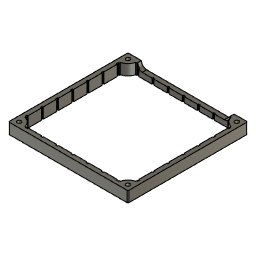
InnerFrame (Autodesk Fusion 360 design; units mm, degrees)
Autodesk Fusion 360 part; units mm, degrees
ref_plane "WorkPlane1" through (0, 0, 36) normal (0, 0, 1) x (1, 0, 0)
sketch "Sketch1" plane through (0, 0, 36) normal (0, 0, 1) x (1, 0, 0)
  line L0 (34, -34) -> (-34, -34)
  line L1 (-34, -34) -> (-34, 34)
  line L2 (-34, 34) -> (34, 34)
  line L3 (34, 34) -> (34, -34)
  line L4 (34, -34) -> (-34, 34) construction
  line L5 (-34, -34) -> (34, 34) construction
  line L6 (-34, 25.5) -> (34, 25.5)
  line L7 (-34, 17) -> (34, 17)
  line L8 (-34, 8.5) -> (34, 8.5)
  line L9 (-34, 0) -> (34, 0)
  line L10 (-25.5, -34) -> (-25.5, 34)
  line L11 (-17, -34) -> (-17, 34)
  line L12 (-8.5, -34) -> (-8.5, 34)
  line L13 (0, -34) -> (0, 34)
  line L14 (-34, 25.5) -> (-25.5, 34) construction
  line L15 (-34, -8.5) -> (34, -8.5)
  line L16 (-34, -17) -> (34, -17)
  line L17 (-34, -25.5) -> (34, -25.5)
  line L18 (-34, -34) -> (34, -34)
  line L19 (8.5, -34) -> (8.5, 34)
  line L20 (17, -34) -> (17, 34)
  line L21 (25.5, -34) -> (25.5, 34)
  line L22 (34, -34) -> (34, 34)
  line L23 (-26.75, 26.75) -> (-32.75, 26.75)
  line L24 (-32.75, 26.75) -> (-32.75, 32.75)
  line L25 (-32.75, 32.75) -> (-26.75, 32.75)
  line L26 (-26.75, 32.75) -> (-26.75, 26.75)
  line L27 (-26.75, 26.75) -> (-32.75, 32.75) construction
  line L28 (-32.75, 26.75) -> (-26.75, 32.75) construction
  line L29 (-24.25, 32.75) -> (-18.25, 32.75)
  line L30 (-24.25, 26.75) -> (-24.25, 32.75)
  line L31 (-18.25, 32.75) -> (-18.25, 26.75)
  line L32 (-18.25, 26.75) -> (-24.25, 26.75)
  line L33 (-15.75, 32.75) -> (-9.75, 32.75)
  line L34 (-15.75, 26.75) -> (-15.75, 32.75)
  line L35 (-9.75, 32.75) -> (-9.75, 26.75)
  line L36 (-9.75, 26.75) -> (-15.75, 26.75)
  line L37 (-7.25, 32.75) -> (-1.25, 32.75)
  line L38 (-7.25, 26.75) -> (-7.25, 32.75)
  line L39 (-1.25, 32.75) -> (-1.25, 26.75)
  line L40 (-1.25, 26.75) -> (-7.25, 26.75)
  line L41 (1.25, 32.75) -> (7.25, 32.75)
  line L42 (1.25, 26.75) -> (1.25, 32.75)
  line L43 (7.25, 32.75) -> (7.25, 26.75)
  line L44 (7.25, 26.75) -> (1.25, 26.75)
  line L45 (9.75, 32.75) -> (15.75, 32.75)
  line L46 (9.75, 26.75) -> (9.75, 32.75)
  line L47 (15.75, 32.75) -> (15.75, 26.75)
  line L48 (15.75, 26.75) -> (9.75, 26.75)
  line L49 (18.25, 32.75) -> (24.25, 32.75)
  line L50 (18.25, 26.75) -> (18.25, 32.75)
  line L51 (24.25, 32.75) -> (24.25, 26.75)
  line L52 (24.25, 26.75) -> (18.25, 26.75)
  line L53 (26.75, 32.75) -> (32.75, 32.75)
  line L54 (26.75, 26.75) -> (26.75, 32.75)
  line L55 (32.75, 32.75) -> (32.75, 26.75)
  line L56 (32.75, 26.75) -> (26.75, 26.75)
  line L57 (-32.75, 24.25) -> (-26.75, 24.25)
  line L58 (-32.75, 18.25) -> (-32.75, 24.25)
  line L59 (-26.75, 24.25) -> (-26.75, 18.25)
  line L60 (-26.75, 18.25) -> (-32.75, 18.25)
  line L61 (-24.25, 24.25) -> (-18.25, 24.25)
  line L62 (-24.25, 18.25) -> (-24.25, 24.25)
  line L63 (-18.25, 24.25) -> (-18.25, 18.25)
  line L64 (-18.25, 18.25) -> (-24.25, 18.25)
  line L65 (-15.75, 24.25) -> (-9.75, 24.25)
  line L66 (-15.75, 18.25) -> (-15.75, 24.25)
  line L67 (-9.75, 24.25) -> (-9.75, 18.25)
  line L68 (-9.75, 18.25) -> (-15.75, 18.25)
  line L69 (-7.25, 24.25) -> (-1.25, 24.25)
  line L70 (-7.25, 18.25) -> (-7.25, 24.25)
  line L71 (-1.25, 24.25) -> (-1.25, 18.25)
  line L72 (-1.25, 18.25) -> (-7.25, 18.25)
  line L73 (1.25, 24.25) -> (7.25, 24.25)
  line L74 (1.25, 18.25) -> (1.25, 24.25)
  line L75 (7.25, 24.25) -> (7.25, 18.25)
  line L76 (7.25, 18.25) -> (1.25, 18.25)
  line L77 (9.75, 24.25) -> (15.75, 24.25)
  line L78 (9.75, 18.25) -> (9.75, 24.25)
  line L79 (15.75, 24.25) -> (15.75, 18.25)
  line L80 (15.75, 18.25) -> (9.75, 18.25)
  line L81 (18.25, 24.25) -> (24.25, 24.25)
  line L82 (18.25, 18.25) -> (18.25, 24.25)
  line L83 (24.25, 24.25) -> (24.25, 18.25)
  line L84 (24.25, 18.25) -> (18.25, 18.25)
  line L85 (26.75, 24.25) -> (32.75, 24.25)
  line L86 (26.75, 18.25) -> (26.75, 24.25)
  line L87 (32.75, 24.25) -> (32.75, 18.25)
  line L88 (32.75, 18.25) -> (26.75, 18.25)
  line L89 (-32.75, 15.75) -> (-26.75, 15.75)
  line L90 (-32.75, 9.75) -> (-32.75, 15.75)
  line L91 (-26.75, 15.75) -> (-26.75, 9.75)
  line L92 (-26.75, 9.75) -> (-32.75, 9.75)
  line L93 (-24.25, 15.75) -> (-18.25, 15.75)
  line L94 (-24.25, 9.75) -> (-24.25, 15.75)
  line L95 (-18.25, 15.75) -> (-18.25, 9.75)
  line L96 (-18.25, 9.75) -> (-24.25, 9.75)
  line L97 (-15.75, 15.75) -> (-9.75, 15.75)
  line L98 (-15.75, 9.75) -> (-15.75, 15.75)
  line L99 (-9.75, 15.75) -> (-9.75, 9.75)
  line L100 (-9.75, 9.75) -> (-15.75, 9.75)
  line L101 (-7.25, 15.75) -> (-1.25, 15.75)
  line L102 (-7.25, 9.75) -> (-7.25, 15.75)
  line L103 (-1.25, 15.75) -> (-1.25, 9.75)
  line L104 (-1.25, 9.75) -> (-7.25, 9.75)
  line L105 (1.25, 15.75) -> (7.25, 15.75)
  line L106 (1.25, 9.75) -> (1.25, 15.75)
  line L107 (7.25, 15.75) -> (7.25, 9.75)
  line L108 (7.25, 9.75) -> (1.25, 9.75)
  line L109 (9.75, 15.75) -> (15.75, 15.75)
  line L110 (9.75, 9.75) -> (9.75, 15.75)
  line L111 (15.75, 15.75) -> (15.75, 9.75)
  line L112 (15.75, 9.75) -> (9.75, 9.75)
  line L113 (18.25, 15.75) -> (24.25, 15.75)
  line L114 (18.25, 9.75) -> (18.25, 15.75)
  line L115 (24.25, 15.75) -> (24.25, 9.75)
  line L116 (24.25, 9.75) -> (18.25, 9.75)
  line L117 (26.75, 15.75) -> (32.75, 15.75)
  line L118 (26.75, 9.75) -> (26.75, 15.75)
  line L119 (32.75, 15.75) -> (32.75, 9.75)
  line L120 (32.75, 9.75) -> (26.75, 9.75)
  line L121 (-32.75, 7.25) -> (-26.75, 7.25)
  line L122 (-32.75, 1.25) -> (-32.75, 7.25)
  line L123 (-26.75, 7.25) -> (-26.75, 1.25)
  line L124 (-26.75, 1.25) -> (-32.75, 1.25)
  line L125 (-24.25, 7.25) -> (-18.25, 7.25)
  line L126 (-24.25, 1.25) -> (-24.25, 7.25)
  line L127 (-18.25, 7.25) -> (-18.25, 1.25)
  line L128 (-18.25, 1.25) -> (-24.25, 1.25)
  line L129 (-15.75, 7.25) -> (-9.75, 7.25)
  line L130 (-15.75, 1.25) -> (-15.75, 7.25)
  line L131 (-9.75, 7.25) -> (-9.75, 1.25)
  line L132 (-9.75, 1.25) -> (-15.75, 1.25)
  line L133 (-7.25, 7.25) -> (-1.25, 7.25)
  line L134 (-7.25, 1.25) -> (-7.25, 7.25)
  line L135 (-1.25, 7.25) -> (-1.25, 1.25)
  line L136 (-1.25, 1.25) -> (-7.25, 1.25)
  line L137 (1.25, 7.25) -> (7.25, 7.25)
  line L138 (1.25, 1.25) -> (1.25, 7.25)
  line L139 (7.25, 7.25) -> (7.25, 1.25)
  line L140 (7.25, 1.25) -> (1.25, 1.25)
  line L141 (9.75, 7.25) -> (15.75, 7.25)
  line L142 (9.75, 1.25) -> (9.75, 7.25)
  line L143 (15.75, 7.25) -> (15.75, 1.25)
  line L144 (15.75, 1.25) -> (9.75, 1.25)
  line L145 (18.25, 7.25) -> (24.25, 7.25)
  line L146 (18.25, 1.25) -> (18.25, 7.25)
  line L147 (24.25, 7.25) -> (24.25, 1.25)
  line L148 (24.25, 1.25) -> (18.25, 1.25)
  line L149 (26.75, 7.25) -> (32.75, 7.25)
  line L150 (26.75, 1.25) -> (26.75, 7.25)
  line L151 (32.75, 7.25) -> (32.75, 1.25)
  line L152 (32.75, 1.25) -> (26.75, 1.25)
  line L153 (-32.75, -1.25) -> (-26.75, -1.25)
  line L154 (-32.75, -7.25) -> (-32.75, -1.25)
  line L155 (-26.75, -1.25) -> (-26.75, -7.25)
  line L156 (-26.75, -7.25) -> (-32.75, -7.25)
  line L157 (-24.25, -1.25) -> (-18.25, -1.25)
  line L158 (-24.25, -7.25) -> (-24.25, -1.25)
  line L159 (-18.25, -1.25) -> (-18.25, -7.25)
  line L160 (-18.25, -7.25) -> (-24.25, -7.25)
  line L161 (-15.75, -1.25) -> (-9.75, -1.25)
  line L162 (-15.75, -7.25) -> (-15.75, -1.25)
  line L163 (-9.75, -1.25) -> (-9.75, -7.25)
  line L164 (-9.75, -7.25) -> (-15.75, -7.25)
  line L165 (-7.25, -1.25) -> (-1.25, -1.25)
  line L166 (-7.25, -7.25) -> (-7.25, -1.25)
  line L167 (-1.25, -1.25) -> (-1.25, -7.25)
  line L168 (-1.25, -7.25) -> (-7.25, -7.25)
  line L169 (1.25, -1.25) -> (7.25, -1.25)
  line L170 (1.25, -7.25) -> (1.25, -1.25)
  line L171 (7.25, -1.25) -> (7.25, -7.25)
  line L172 (7.25, -7.25) -> (1.25, -7.25)
  line L173 (9.75, -1.25) -> (15.75, -1.25)
  line L174 (9.75, -7.25) -> (9.75, -1.25)
  line L175 (15.75, -1.25) -> (15.75, -7.25)
  line L176 (15.75, -7.25) -> (9.75, -7.25)
  line L177 (18.25, -1.25) -> (24.25, -1.25)
  line L178 (18.25, -7.25) -> (18.25, -1.25)
  line L179 (24.25, -1.25) -> (24.25, -7.25)
  line L180 (24.25, -7.25) -> (18.25, -7.25)
  line L181 (26.75, -1.25) -> (32.75, -1.25)
  line L182 (26.75, -7.25) -> (26.75, -1.25)
  line L183 (32.75, -1.25) -> (32.75, -7.25)
  line L184 (32.75, -7.25) -> (26.75, -7.25)
  line L185 (-32.75, -9.75) -> (-26.75, -9.75)
  line L186 (-32.75, -15.75) -> (-32.75, -9.75)
  line L187 (-26.75, -9.75) -> (-26.75, -15.75)
  line L188 (-26.75, -15.75) -> (-32.75, -15.75)
  line L189 (-24.25, -9.75) -> (-18.25, -9.75)
  line L190 (-24.25, -15.75) -> (-24.25, -9.75)
  line L191 (-18.25, -9.75) -> (-18.25, -15.75)
  line L192 (-18.25, -15.75) -> (-24.25, -15.75)
  line L193 (-15.75, -9.75) -> (-9.75, -9.75)
  line L194 (-15.75, -15.75) -> (-15.75, -9.75)
  line L195 (-9.75, -9.75) -> (-9.75, -15.75)
  line L196 (-9.75, -15.75) -> (-15.75, -15.75)
  line L197 (-7.25, -9.75) -> (-1.25, -9.75)
  line L198 (-7.25, -15.75) -> (-7.25, -9.75)
  line L199 (-1.25, -9.75) -> (-1.25, -15.75)
  line L200 (-1.25, -15.75) -> (-7.25, -15.75)
  line L201 (1.25, -9.75) -> (7.25, -9.75)
  line L202 (1.25, -15.75) -> (1.25, -9.75)
  line L203 (7.25, -9.75) -> (7.25, -15.75)
  line L204 (7.25, -15.75) -> (1.25, -15.75)
  line L205 (9.75, -9.75) -> (15.75, -9.75)
  line L206 (9.75, -15.75) -> (9.75, -9.75)
  line L207 (15.75, -9.75) -> (15.75, -15.75)
  line L208 (15.75, -15.75) -> (9.75, -15.75)
  line L209 (18.25, -9.75) -> (24.25, -9.75)
  line L210 (18.25, -15.75) -> (18.25, -9.75)
  line L211 (24.25, -9.75) -> (24.25, -15.75)
  line L212 (24.25, -15.75) -> (18.25, -15.75)
  line L213 (26.75, -9.75) -> (32.75, -9.75)
  line L214 (26.75, -15.75) -> (26.75, -9.75)
  line L215 (32.75, -9.75) -> (32.75, -15.75)
  line L216 (32.75, -15.75) -> (26.75, -15.75)
  line L217 (-32.75, -18.25) -> (-26.75, -18.25)
  line L218 (-32.75, -24.25) -> (-32.75, -18.25)
  line L219 (-26.75, -18.25) -> (-26.75, -24.25)
  line L220 (-26.75, -24.25) -> (-32.75, -24.25)
  line L221 (-24.25, -18.25) -> (-18.25, -18.25)
  line L222 (-24.25, -24.25) -> (-24.25, -18.25)
  line L223 (-18.25, -18.25) -> (-18.25, -24.25)
  line L224 (-18.25, -24.25) -> (-24.25, -24.25)
  line L225 (-15.75, -18.25) -> (-9.75, -18.25)
  line L226 (-15.75, -24.25) -> (-15.75, -18.25)
  line L227 (-9.75, -18.25) -> (-9.75, -24.25)
  line L228 (-9.75, -24.25) -> (-15.75, -24.25)
  line L229 (-7.25, -18.25) -> (-1.25, -18.25)
  line L230 (-7.25, -24.25) -> (-7.25, -18.25)
  line L231 (-1.25, -18.25) -> (-1.25, -24.25)
  line L232 (-1.25, -24.25) -> (-7.25, -24.25)
  line L233 (1.25, -18.25) -> (7.25, -18.25)
  line L234 (1.25, -24.25) -> (1.25, -18.25)
  line L235 (7.25, -18.25) -> (7.25, -24.25)
  line L236 (7.25, -24.25) -> (1.25, -24.25)
  line L237 (9.75, -18.25) -> (15.75, -18.25)
  line L238 (9.75, -24.25) -> (9.75, -18.25)
  line L239 (15.75, -18.25) -> (15.75, -24.25)
  line L240 (15.75, -24.25) -> (9.75, -24.25)
  line L241 (18.25, -18.25) -> (24.25, -18.25)
  line L242 (18.25, -24.25) -> (18.25, -18.25)
  line L243 (24.25, -18.25) -> (24.25, -24.25)
  line L244 (24.25, -24.25) -> (18.25, -24.25)
  line L245 (26.75, -18.25) -> (32.75, -18.25)
  line L246 (26.75, -24.25) -> (26.75, -18.25)
  line L247 (32.75, -18.25) -> (32.75, -24.25)
  line L248 (32.75, -24.25) -> (26.75, -24.25)
  line L249 (-32.75, -26.75) -> (-26.75, -26.75)
  line L250 (-32.75, -32.75) -> (-32.75, -26.75)
  line L251 (-26.75, -26.75) -> (-26.75, -32.75)
  line L252 (-26.75, -32.75) -> (-32.75, -32.75)
  line L253 (-24.25, -26.75) -> (-18.25, -26.75)
  line L254 (-24.25, -32.75) -> (-24.25, -26.75)
  line L255 (-18.25, -26.75) -> (-18.25, -32.75)
  line L256 (-18.25, -32.75) -> (-24.25, -32.75)
  line L257 (-15.75, -26.75) -> (-9.75, -26.75)
  line L258 (-15.75, -32.75) -> (-15.75, -26.75)
  line L259 (-9.75, -26.75) -> (-9.75, -32.75)
  line L260 (-9.75, -32.75) -> (-15.75, -32.75)
  line L261 (-7.25, -26.75) -> (-1.25, -26.75)
  line L262 (-7.25, -32.75) -> (-7.25, -26.75)
  line L263 (-1.25, -26.75) -> (-1.25, -32.75)
  line L264 (-1.25, -32.75) -> (-7.25, -32.75)
  line L265 (1.25, -26.75) -> (7.25, -26.75)
  line L266 (1.25, -32.75) -> (1.25, -26.75)
  line L267 (7.25, -26.75) -> (7.25, -32.75)
  line L268 (7.25, -32.75) -> (1.25, -32.75)
  line L269 (9.75, -26.75) -> (15.75, -26.75)
  line L270 (9.75, -32.75) -> (9.75, -26.75)
  line L271 (15.75, -26.75) -> (15.75, -32.75)
  line L272 (15.75, -32.75) -> (9.75, -32.75)
  line L273 (18.25, -26.75) -> (24.25, -26.75)
  line L274 (18.25, -32.75) -> (18.25, -26.75)
  line L275 (24.25, -26.75) -> (24.25, -32.75)
  line L276 (24.25, -32.75) -> (18.25, -32.75)
  line L277 (26.75, -26.75) -> (32.75, -26.75)
  line L278 (26.75, -32.75) -> (26.75, -26.75)
  line L279 (32.75, -26.75) -> (32.75, -32.75)
  line L280 (32.75, -32.75) -> (26.75, -32.75)
  line L281 (36, -36) -> (-36, -36)
  line L282 (-36, -36) -> (-36, 36)
  line L283 (-36, 36) -> (36, 36)
  line L284 (36, 36) -> (36, -36)
  line L285 (36, -36) -> (-36, 36) construction
  line L286 (-36, -36) -> (36, 36) construction
  line L287 (0.8, -34) -> (0.8, 34)
  line L288 (9.3, -34) -> (9.3, 34)
  line L289 (17.8, -34) -> (17.8, 34)
  line L290 (26.3, -34) -> (26.3, 34)
  line L291 (33.2, 34) -> (33.2, -34)
  line L292 (34.8, 34) -> (34.8, -34)
  line L293 (24.7, -34) -> (24.7, 34)
  line L294 (16.2, -34) -> (16.2, 34)
  line L295 (7.7, -34) -> (7.7, 34)
  line L296 (-0.8, -34) -> (-0.8, 34)
  line L297 (-34, -26.3) -> (34, -26.3)
  line L298 (-34, -24.7) -> (34, -24.7)
  line L299 (-34, -17.8) -> (34, -17.8)
  line L300 (-34, -16.2) -> (34, -16.2)
  line L301 (-34, -9.3) -> (34, -9.3)
  line L302 (-34, -7.7) -> (34, -7.7)
  line L303 (-34, -0.8) -> (34, -0.8)
  line L304 (-34, 0.8) -> (34, 0.8)
  line L305 (-7.7, -34) -> (-7.7, 34)
  line L306 (-9.3, -34) -> (-9.3, 34)
  line L307 (-16.2, -34) -> (-16.2, 34)
  line L308 (-17.8, -34) -> (-17.8, 34)
  line L309 (-24.7, -34) -> (-24.7, 34)
  line L310 (-26.3, -34) -> (-26.3, 34)
  line L311 (-33.2, -34) -> (-33.2, 34)
  line L312 (-34.8, -34) -> (-34.8, 34)
  line L313 (34, -33.2) -> (-34, -33.2)
  line L314 (33.2, -33.2) -> (-33.2, -33.2)
  line L315 (-33.2, -33.2) -> (-33.2, 33.2)
  line L316 (-33.2, 33.2) -> (33.2, 33.2)
  line L317 (33.2, 33.2) -> (33.2, -33.2)
  point P0 (-29.75, 29.75)
  dimension "d701_1_2" = 68
  dimension "d702_1_2" = 68
  dimension "d705_1_2" = 0
  dimension "d706_1_2" = -68
  dimension "d709_1_2" = 68
  dimension "d710_1_2" = 0
  dimension "d711_1_2" = 6
  dimension "d712_1_2" = 6
  dimension "d715_1_2" = 8.5
  dimension "d716_1_2" = -8.5
  dimension "d718_1_2" = 72
  dimension "d719_1_2" = 72
  dimension "d815_2" = 0.8
  dimension "d816_2" = 0.8
  dimension "d817_2" = 0.8
  dimension "d818_2" = 0.8
  dimension "d819_2" = 0.8
  dimension "d825_2" = 0.8
  dimension "d827_2" = 0.8
  dimension "d829_2" = 0.8
  dimension "d831_2" = 0.8
  dimension "d833_2" = 0.8
  dimension "d835_2" = 0.8
  dimension "d837_2" = 0.8
  dimension "d839_2" = 0.8
  dimension "d841_2" = 0.8
  dimension "d1156" = 0.8
  constraint horizontal L0
  constraint perpendicular L0 L1
  constraint parallel L0 L2
  constraint parallel L1 L3
  constraint coincident L4 origin
  constraint coincident L5 origin
  constraint horizontal L23
  constraint perpendicular L23 L24
  constraint parallel L23 L25
  constraint parallel L24 L26
  constraint coincident L27 P0
  constraint coincident L28 P0
  constraint midpoint L14 P0
  constraint horizontal L281
  constraint perpendicular L281 L282
  constraint parallel L281 L283
  constraint parallel L282 L284
  constraint coincident L285 origin
  constraint coincident L286 origin
  measures "d701_1_2" distance of L1.end L2.end
  measures "d702_1_2" distance of L0.end L1.end
  measures "d711_1_2" distance of L24.end L25.end
  measures "d712_1_2" distance of L23.end L24.end
  measures "d718_1_2" distance of L282.end L283.end
  measures "d719_1_2" distance of L281.end L282.end
sketch "Sketch54" plane through (0, 0, 36) normal (0, 0, 1) x (1, 0, 0)
  line L0 (34, -34) -> (-34, -34)
  line L1 (-34, -34) -> (-34, 34)
  line L2 (-34, 34) -> (34, 34)
  line L3 (34, 34) -> (34, -34)
  line L4 (34, -34) -> (-34, 34) construction
  line L5 (-34, -34) -> (34, 34) construction
  line L6 (33.5, -33.5) -> (-33.5, -33.5)
  line L7 (-33.5, -33.5) -> (-33.5, 33.5)
  line L8 (-33.5, 33.5) -> (33.5, 33.5)
  line L9 (33.5, 33.5) -> (33.5, -33.5)
  line L10 (-32.5, -32.5) -> (-32.5, 32.5)
  line L11 (-32.5, 32.5) -> (32.5, 32.5)
  line L12 (32.5, 32.5) -> (32.5, -32.5)
  line L13 (32.5, -32.5) -> (-32.5, -32.5)
  line L14 (-34, 25.5) -> (34, 25.5) construction
  line L15 (-34, 17) -> (34, 17) construction
  line L16 (-34, 8.5) -> (34, 8.5) construction
  line L17 (-34, 0) -> (34, 0) construction
  line L18 (-34, -8.5) -> (34, -8.5) construction
  line L19 (-34, -17) -> (34, -17) construction
  line L20 (-34, -25.5) -> (34, -25.5) construction
  line L21 (-34, -34) -> (34, -34)
  line L22 (-25.5, -34) -> (-25.5, 34) construction
  line L23 (-17, -34) -> (-17, 34) construction
  line L24 (-8.5, -34) -> (-8.5, 34) construction
  line L25 (0, -34) -> (0, 34) construction
  line L26 (8.5, -34) -> (8.5, 34) construction
  line L27 (17, -34) -> (17, 34) construction
  line L28 (25.5, -34) -> (25.5, 34) construction
  line L29 (34, -34) -> (34, 34)
  arc A0 (-26.5, -32.5) -> (-32.5, -26.5) centre (-32.5, -32.5) ccw
  arc A1 (-32.5, 26.5) -> (-26.5, 32.5) centre (-32.5, 32.5) ccw
  arc A2 (26.5, 32.5) -> (32.5, 26.5) centre (32.5, 32.5) ccw
  arc A3 (32.5, -26.5) -> (26.5, -32.5) centre (32.5, -32.5) ccw
  circle A4 centre (-30.5, 30.5) radius 1.1
  circle A5 centre (30.5, 30.5) radius 1.1
  circle A6 centre (-30.5, -30.5) radius 1.1
  circle A7 centre (30.5, -30.5) radius 1.1
  line L30 (-32.5, 17) -> (-32.5, 19)
  line L31 (-31, 19) -> (-31, 0)
  line L32 (-32.5, 17) -> (-32.5, 17.5)
  line L33 (-32.5, 17) -> (-32.5, 16.5)
  line L34 (-32.5, 8.5) -> (-32.5, 9)
  line L35 (-32.5, 8.5) -> (-32.5, 8)
  line L36 (-31, -19) -> (-31, 0)
  line L37 (-19, -31) -> (0, -31)
  line L38 (19, -31) -> (0, -31)
  line L39 (31, -19) -> (31, 0)
  line L40 (31, 19) -> (31, 0)
  line L41 (19, 31) -> (0, 31)
  line L42 (-19, 31) -> (0, 31)
  line L43 (31, 0) -> (31, 0.5)
  line L44 (31, 0) -> (31, -0.5)
  line L45 (31, 19) -> (31, 26.6905)
  line L46 (19, 31) -> (26.6905, 31)
  line L47 (-19, 31) -> (-26.6905, 31)
  line L48 (-31, 19) -> (-31, 26.6905)
  line L49 (-31, -19) -> (-31, -26.6905)
  line L50 (19, -31) -> (26.6905, -31)
  line L51 (-19, -31) -> (-26.6905, -31)
  line L52 (31, -19) -> (31, -26.6905)
  line L53 (-31, 25.5) -> (-31, 26)
  line L54 (-31, 26) -> (-31.5, 26)
  line L55 (-31.5, 26) -> (-31.5, 25)
  line L56 (-31.5, 25) -> (-31, 25)
  line L57 (-31, 17.5) -> (-31.5, 17.5)
  line L58 (-31.5, 17.5) -> (-31.5, 16.5)
  line L59 (-31.5, 16.5) -> (-31, 16.5)
  line L60 (-31, 9) -> (-31.5, 9)
  line L61 (-31.5, 9) -> (-31.5, 8)
  line L62 (-31.5, 8) -> (-31, 8)
  line L63 (-31, 0.5) -> (-31.5, 0.5)
  line L64 (-31.5, 0.5) -> (-31.5, -0.5)
  line L65 (-31.5, -0.5) -> (-31, -0.5)
  line L66 (-31, -8) -> (-31.5, -8)
  line L67 (-31.5, -8) -> (-31.5, -9)
  line L68 (-31.5, -9) -> (-31, -9)
  line L69 (-31, -16.5) -> (-31.5, -16.5)
  line L70 (-31.5, -16.5) -> (-31.5, -17.5)
  line L71 (-31.5, -17.5) -> (-31, -17.5)
  line L72 (-31, -25) -> (-31.5, -25)
  line L73 (-31.5, -25) -> (-31.5, -26)
  line L74 (-31.5, -26) -> (-31, -26)
  line L75 (-26, -31.5) -> (-25, -31.5)
  line L76 (-25, -31.5) -> (-25, -31)
  line L77 (-26, -31) -> (-26, -31.5)
  line L78 (-17.5, -31) -> (-17.5, -31.5)
  line L79 (-17.5, -31.5) -> (-16.5, -31.5)
  line L80 (-16.5, -31.5) -> (-16.5, -31)
  line L81 (-9, -31) -> (-9, -31.5)
  line L82 (-9, -31.5) -> (-8, -31.5)
  line L83 (-8, -31.5) -> (-8, -31)
  line L84 (-0.5, -31) -> (-0.5, -31.5)
  line L85 (-0.5, -31.5) -> (0.5, -31.5)
  line L86 (0.5, -31.5) -> (0.5, -31)
  line L87 (8, -31) -> (8, -31.5)
  line L88 (8, -31.5) -> (9, -31.5)
  line L89 (9, -31.5) -> (9, -31)
  line L90 (16.5, -31) -> (16.5, -31.5)
  line L91 (16.5, -31.5) -> (17.5, -31.5)
  line L92 (17.5, -31.5) -> (17.5, -31)
  line L93 (25, -31) -> (25, -31.5)
  line L94 (25, -31.5) -> (26, -31.5)
  line L95 (26, -31.5) -> (26, -31)
  line L96 (31.5, -26) -> (31.5, -25)
  line L97 (31.5, -25) -> (31, -25)
  line L98 (31, -26) -> (31.5, -26)
  line L99 (31, -17.5) -> (31.5, -17.5)
  line L100 (31.5, -17.5) -> (31.5, -16.5)
  line L101 (31.5, -16.5) -> (31, -16.5)
  line L102 (31, -9) -> (31.5, -9)
  line L103 (31.5, -9) -> (31.5, -8)
  line L104 (31.5, -8) -> (31, -8)
  line L105 (31, -0.5) -> (31.5, -0.5)
  line L106 (31.5, -0.5) -> (31.5, 0.5)
  line L107 (31.5, 0.5) -> (31, 0.5)
  line L108 (31, 8) -> (31.5, 8)
  line L109 (31.5, 8) -> (31.5, 9)
  line L110 (31.5, 9) -> (31, 9)
  line L111 (31, 16.5) -> (31.5, 16.5)
  line L112 (31.5, 16.5) -> (31.5, 17.5)
  line L113 (31.5, 17.5) -> (31, 17.5)
  line L114 (31, 25) -> (31.5, 25)
  line L115 (31.5, 25) -> (31.5, 26)
  line L116 (31.5, 26) -> (31, 26)
  line L117 (26, 31.5) -> (25, 31.5)
  line L118 (25, 31.5) -> (25, 31)
  line L119 (26, 31) -> (26, 31.5)
  line L120 (17.5, 31) -> (17.5, 31.5)
  line L121 (17.5, 31.5) -> (16.5, 31.5)
  line L122 (16.5, 31.5) -> (16.5, 31)
  line L123 (9, 31) -> (9, 31.5)
  line L124 (9, 31.5) -> (8, 31.5)
  line L125 (8, 31.5) -> (8, 31)
  line L126 (0.5, 31) -> (0.5, 31.5)
  line L127 (0.5, 31.5) -> (-0.5, 31.5)
  line L128 (-0.5, 31.5) -> (-0.5, 31)
  line L129 (-8, 31) -> (-8, 31.5)
  line L130 (-8, 31.5) -> (-9, 31.5)
  line L131 (-9, 31.5) -> (-9, 31)
  line L132 (-16.5, 31) -> (-16.5, 31.5)
  line L133 (-16.5, 31.5) -> (-17.5, 31.5)
  line L134 (-17.5, 31.5) -> (-17.5, 31)
  line L135 (-25, 31) -> (-25, 31.5)
  line L136 (-25, 31.5) -> (-26, 31.5)
  line L137 (-26, 31.5) -> (-26, 31)
  dimension "d1157" = 68
  dimension "d1158" = 68
  dimension "d1159" = 0.5
  dimension "d1160" = 1.5
  dimension "d1163" = 0
  dimension "d1164" = -68
  dimension "d1167" = 68
  dimension "d1168" = 0
  dimension "d1171" = 6
  dimension "d1172" = 6
  dimension "d1173" = 6
  dimension "d1174" = 6
  dimension "d1175" = 2.2
  dimension "d1182" = 1.5
  dimension "d1197" = 8.5
  dimension "d1198" = -8.5
  dimension "d1200" = 360
  constraint horizontal L0
  constraint perpendicular L0 L1
  constraint parallel L0 L2
  constraint parallel L1 L3
  constraint coincident L4 origin
  constraint coincident L5 origin
  constraint coincident L13 A0.start
  constraint coincident L10.start L13.end
  constraint coincident L10.end L11.start
  constraint coincident L11.end L12.start
  constraint coincident L12 A3.start
  constraint coincident L12.end L13.start
  constraint coincident L4 A4.centre
  constraint symmetric L25 A4 A5
  constraint symmetric L17 A4 A6
  constraint symmetric L17 A5 A7
  constraint coincident L10 L30.start
  constraint coincident L15 L30.start
  constraint coincident L10 L30.end
  constraint perpendicular L15 L30
  constraint coincident L17 L31.end
  constraint perpendicular L17 L31
  constraint coincident L30 L32.end
  constraint coincident L10 L33.end
  constraint coincident L10 L34.start
  constraint coincident L16 L34.start
  constraint coincident L10 L34.end
  constraint coincident L10 L35.end
  constraint symmetric L17 L31.start L36.start
  constraint symmetric L17 L31.end L36.end
  constraint coincident L40 L43.end
  constraint coincident L39 L44.end
  constraint coincident A2 L45.end
  constraint perpendicular L14 L45
  constraint coincident A2 L46.end
  constraint perpendicular L28 L46
  constraint coincident A1 L47.end
  constraint coincident A1 L48.end
  constraint perpendicular L14 L48
  constraint coincident A0 L49.end
  constraint coincident A3 L50.end
  constraint perpendicular L28 L50
  constraint coincident A0 L51.end
  constraint perpendicular L22 L51
  constraint coincident A3 L52.end
  constraint perpendicular L20 L52
  constraint coincident L48 L53.start
  constraint coincident L14 L53.start
  constraint coincident L48 L53.end
  constraint perpendicular L53 L54
  constraint perpendicular L14 L55
  constraint coincident L48 L56.end
  constraint perpendicular L48 L56
  measures "d1157" distance of L1.end L2.end
  measures "d1158" distance of L0.end L1.end
  measures "d1171" radius of A0
  measures "d1172" radius of A1
  measures "d1173" radius of A2
  measures "d1174" radius of A3
  measures "d1175" diameter of A4
  measures "d1182" distance of L30.end L31.start
extrude "Extrude8" add sketch "Sketch54" along normal blind 6 contours L6 L7 L8 L9
extrude "Extrude9" add sketch "Sketch54" along normal blind 6 contours L10 L13 A0 | L12 L13 A3 | L11 L12 A2 | L10 L11 A1
fillet "Fillet2" radius 0.5 4 edges at (-33.5, 33.5, 39) (-33.5, -33.5, 39) (33.5, 33.5, 39) (33.5, -33.5, 39)
extrude "Extrude11" add sketch "Sketch54" along normal blind 6 contours L10 A0 A1 L30 L31 L32 L33 L34 L35 L36 L48 L49 L54 L55 L56 L57 L58 L59 L60 L61 L62 L63 L64 L65 L66 L67 L68 L69 L70 L71 L72 L73 L74 | L13 A0 A3 L37 L38 L50 L51 L75 L76 L77 L78 L79 L80 L81 L82 L83 L84 L85 L86 L87 L88 L89 L90 L91 L92 L93 L94 L95 | L12 A2 A3 L39 L40 L45 L52 L96 L97 L98 L99 L100 L101 L102 L103 L104 L105 L106 L107 L108 L109 L110 L111 L112 L113 L114 L115 L116 | L11 A1 A2 L41 L42 L46 L47 L117 L118 L119 L120 L121 L122 L123 L124 L125 L126 L127 L128 L129 L130 L131 L132 L133 L134 L135 L136 L137
sketch "Sketch55" plane through (0, 0, 42) normal (0, 0, 1) x (-1, 0, 0)
  arc A0 (-33, 33.5) -> (-33.5, 33) centre (-33, 33) ccw
  line L0 (-33.5, 33) -> (-33.5, -33)
  arc A1 (-33.5, -33) -> (-33, -33.5) centre (-33, -33) ccw
  line L1 (-33, -33.5) -> (33, -33.5)
  arc A2 (33, -33.5) -> (33.5, -33) centre (33, -33) ccw
  line L2 (33.5, -33) -> (33.5, 33)
  arc A3 (33.5, 33) -> (33, 33.5) centre (33, 33) ccw
  line L3 (33, 33.5) -> (-33, 33.5)
  circle A4 centre (-30.5, -30.5) radius 1.1
  circle A5 centre (-30.5, 30.5) radius 1.1
  circle A6 centre (30.5, -30.5) radius 1.1
  circle A7 centre (30.5, 30.5) radius 1.1
  arc A8 (31, -26.6905) -> (26.6905, -31) centre (32.5, -32.5) ccw
  line L4 (26.6905, -31) -> (26, -31)
  line L5 (26, -31) -> (26, -31.5)
  line L6 (26, -31.5) -> (25, -31.5)
  line L7 (25, -31.5) -> (25, -31)
  line L8 (25, -31) -> (17.5, -31)
  line L9 (17.5, -31) -> (17.5, -31.5)
  line L10 (17.5, -31.5) -> (16.5, -31.5)
  line L11 (16.5, -31.5) -> (16.5, -31)
  line L12 (16.5, -31) -> (9, -31)
  line L13 (9, -31) -> (9, -31.5)
  line L14 (9, -31.5) -> (8, -31.5)
  line L15 (8, -31.5) -> (8, -31)
  line L16 (8, -31) -> (0.5, -31)
  line L17 (0.5, -31) -> (0.5, -31.5)
  line L18 (0.5, -31.5) -> (-0.5, -31.5)
  line L19 (-0.5, -31.5) -> (-0.5, -31)
  line L20 (-0.5, -31) -> (-8, -31)
  line L21 (-8, -31) -> (-8, -31.5)
  line L22 (-8, -31.5) -> (-9, -31.5)
  line L23 (-9, -31.5) -> (-9, -31)
  line L24 (-9, -31) -> (-16.5, -31)
  line L25 (-16.5, -31) -> (-16.5, -31.5)
  line L26 (-16.5, -31.5) -> (-17.5, -31.5)
  line L27 (-17.5, -31.5) -> (-17.5, -31)
  line L28 (-17.5, -31) -> (-25, -31)
  line L29 (-25, -31) -> (-25, -31.5)
  line L30 (-25, -31.5) -> (-26, -31.5)
  line L31 (-26, -31.5) -> (-26, -31)
  line L32 (-26, -31) -> (-26.6905, -31)
  arc A9 (-26.6905, -31) -> (-31, -26.6905) centre (-32.5, -32.5) ccw
  line L33 (-31, -26.6905) -> (-31, -26)
  line L34 (-31, -26) -> (-31.5, -26)
  line L35 (-31.5, -26) -> (-31.5, -25)
  line L36 (-31.5, -25) -> (-31, -25)
  line L37 (-31, -25) -> (-31, -17.5)
  line L38 (-31, -17.5) -> (-31.5, -17.5)
  line L39 (-31.5, -17.5) -> (-31.5, -16.5)
  line L40 (-31.5, -16.5) -> (-31, -16.5)
  line L41 (-31, -16.5) -> (-31, -9)
  line L42 (-31, -9) -> (-31.5, -9)
  line L43 (-31.5, -9) -> (-31.5, -8)
  line L44 (-31.5, -8) -> (-31, -8)
  line L45 (-31, -8) -> (-31, -0.5)
  line L46 (-31, -0.5) -> (-31.5, -0.5)
  line L47 (-31.5, -0.5) -> (-31.5, 0.5)
  line L48 (-31.5, 0.5) -> (-31, 0.5)
  line L49 (-31, 0.5) -> (-31, 8)
  line L50 (-31, 8) -> (-31.5, 8)
  line L51 (-31.5, 8) -> (-31.5, 9)
  line L52 (-31.5, 9) -> (-31, 9)
  line L53 (-31, 9) -> (-31, 16.5)
  line L54 (-31, 16.5) -> (-31.5, 16.5)
  line L55 (-31.5, 16.5) -> (-31.5, 17.5)
  line L56 (-31.5, 17.5) -> (-31, 17.5)
  line L57 (-31, 17.5) -> (-31, 25)
  line L58 (-31, 25) -> (-31.5, 25)
  line L59 (-31.5, 25) -> (-31.5, 26)
  line L60 (-31.5, 26) -> (-31, 26)
  line L61 (-31, 26) -> (-31, 26.6905)
  arc A10 (-31, 26.6905) -> (-26.6905, 31) centre (-32.5, 32.5) ccw
  line L62 (-26.6905, 31) -> (-26, 31)
  line L63 (-26, 31) -> (-26, 31.5)
  line L64 (-26, 31.5) -> (-25, 31.5)
  line L65 (-25, 31.5) -> (-25, 31)
  line L66 (-25, 31) -> (-17.5, 31)
  line L67 (-17.5, 31) -> (-17.5, 31.5)
  line L68 (-17.5, 31.5) -> (-16.5, 31.5)
  line L69 (-16.5, 31.5) -> (-16.5, 31)
  line L70 (-16.5, 31) -> (-9, 31)
  line L71 (-9, 31) -> (-9, 31.5)
  line L72 (-9, 31.5) -> (-8, 31.5)
  line L73 (-8, 31.5) -> (-8, 31)
  line L74 (-8, 31) -> (-0.5, 31)
  line L75 (-0.5, 31) -> (-0.5, 31.5)
  line L76 (-0.5, 31.5) -> (0.5, 31.5)
  line L77 (0.5, 31.5) -> (0.5, 31)
  line L78 (0.5, 31) -> (8, 31)
  line L79 (8, 31) -> (8, 31.5)
  line L80 (8, 31.5) -> (9, 31.5)
  line L81 (9, 31.5) -> (9, 31)
  line L82 (9, 31) -> (16.5, 31)
  line L83 (16.5, 31) -> (16.5, 31.5)
  line L84 (16.5, 31.5) -> (17.5, 31.5)
  line L85 (17.5, 31.5) -> (17.5, 31)
  line L86 (17.5, 31) -> (25, 31)
  line L87 (25, 31) -> (25, 31.5)
  line L88 (25, 31.5) -> (26, 31.5)
  line L89 (26, 31.5) -> (26, 31)
  line L90 (26, 31) -> (26.6905, 31)
  arc A11 (26.6905, 31) -> (31, 26.6905) centre (32.5, 32.5) ccw
  line L91 (31, 26.6905) -> (31, 26)
  line L92 (31, 26) -> (31.5, 26)
  line L93 (31.5, 26) -> (31.5, 25)
  line L94 (31.5, 25) -> (31, 25)
  line L95 (31, 25) -> (31, 17.5)
  line L96 (31, 17.5) -> (31.5, 17.5)
  line L97 (31.5, 17.5) -> (31.5, 16.5)
  line L98 (31.5, 16.5) -> (31, 16.5)
  line L99 (31, 16.5) -> (31, 9)
  line L100 (31, 9) -> (31.5, 9)
  line L101 (31.5, 9) -> (31.5, 8)
  line L102 (31.5, 8) -> (31, 8)
  line L103 (31, 8) -> (31, 0.5)
  line L104 (31, 0.5) -> (31.5, 0.5)
  line L105 (31.5, 0.5) -> (31.5, -0.5)
  line L106 (31.5, -0.5) -> (31, -0.5)
  line L107 (31, -0.5) -> (31, -8)
  line L108 (31, -8) -> (31.5, -8)
  line L109 (31.5, -8) -> (31.5, -9)
  line L110 (31.5, -9) -> (31, -9)
  line L111 (31, -9) -> (31, -16.5)
  line L112 (31, -16.5) -> (31.5, -16.5)
  line L113 (31.5, -16.5) -> (31.5, -17.5)
  line L114 (31.5, -17.5) -> (31, -17.5)
  line L115 (31, -17.5) -> (31, -25)
  line L116 (31, -25) -> (31.5, -25)
  line L117 (31.5, -25) -> (31.5, -26)
  line L118 (31.5, -26) -> (31, -26)
  line L119 (31, -26) -> (31, -26.6905)
  line L120 (-26, -31.5) -> (-26, -33.5)
  line L121 (26, -31.5) -> (26, -33.5)
  constraint coincident L30.end L31.start
  constraint coincident L1 L120.end
  constraint perpendicular L1 L120
  constraint coincident L5.end L6.start
  constraint coincident L1 L121.end
  constraint perpendicular L1 L121
extrude "Extrude13" cut sketch "Sketch55" against normal blind 3 contours L1 L6 L7 L8 L9 L10 L11 L12 L13 L14 L15 L16 L17 L18 L19 L20 L21 L22 L23 L24 L25 L26 L27 L28 L29 L30 L120 L121
fillet "Fillet5" radius 3 2 edges at (26, 32.5, 39) (-26, 32.5, 39)
equation "d815_2 = LaserGap"
equation "d816_2 = LaserGap"
equation "d817_2 = LaserGap"
equation "d818_2 = LaserGap"
equation "d819_2 = LaserGap"
equation "d820_2 = -LaserGap"
equation "d821_2 = -LaserGap"
equation "d822_2 = -LaserGap"
equation "d823_2 = -LaserGap"
equation "d824_2 = -LaserGap"
equation "d825_2 = LaserGap"
equation "d826_2 = -LaserGap"
equation "d827_2 = LaserGap"
equation "d828_2 = -LaserGap"
equation "d829_2 = LaserGap"
equation "d830_2 = -LaserGap"
equation "d831_2 = LaserGap"
equation "d832_2 = -LaserGap"
equation "d833_2 = LaserGap"
equation "d834_2 = -LaserGap"
equation "d835_2 = LaserGap"
equation "d836_2 = -LaserGap"
equation "d837_2 = LaserGap"
equation "d838_2 = -LaserGap"
equation "d839_2 = LaserGap"
equation "d840_2 = -LaserGap"
equation "d841_2 = LaserGap"
equation "d1156 = LaserGap"
equation "LaserGap = 0.8 mm"
